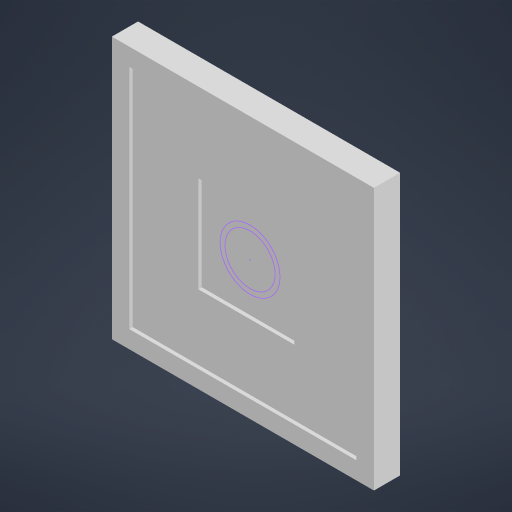
# Autodesk Inventor part: Elbow_Both_Marker_TestFit_V2
Saved by Autodesk Inventor 2024 (Build 280153000, 153)
## iProperties
Created: 2023-06-29
Part Number: Elbow_Both_Marker_TestFit_V2
Material: Generic
Document SubType Name: Modeling
Designer: User
Density: 1 g/cm^3
Appearance: Default
Author: User
Autodesk Inventor part; units mm, degrees
ref_plane "YZ Plane" through (0, 0, 0) normal (1, 0, 0) x (0, 1, 0)
ref_plane "XZ Plane" through (0, 0, 0) normal (0, 1, 0) x (-1, 0, 0)
ref_plane "XY Plane" through (0, 0, 0) normal (0, 0, 1) x (1, 0, 0)
sketch "Sketch4" plane through (0, 0, 0) normal (0, 0, 1) x (1, 0, 0)
  line L0 (0, 0) -> (150, 0)
  line L1 (150, 0) -> (150, 150)
  line L2 (150, 150) -> (0, 150)
  line L3 (0, 150) -> (0, 0)
  dimension "d34" = 150
  dimension "d35" = 150
  constraints: 8 end point, 2 parallel, 1 horizontal, 1 perpendicular
  measures "d34" distance of L2.end L1.end
  measures "d35" distance of L1.end L0.end
extrude "Extrusion4" add sketch "Sketch4" along normal blind 10
sketch "Sketch5" plane through (0, 0, 10) normal (0, 0, 1) x (1, 0, 0)
  line L0 (10, 10) -> (140, 10)
  line L1 (140, 10) -> (140, 140)
  line L2 (140, 140) -> (10, 140)
  line L3 (10, 140) -> (10, 10)
  point P0 (0, 0)
  dimension "d38" = 130
  dimension "d39" = 130
  constraints: 8 end point, 2 parallel, 1 horizontal, 1 perpendicular
  measures "d38" distance of L2.end L1.end
  measures "d39" distance of L1.end L0.end
extrude "Extrusion5" cut sketch "Sketch5" against normal blind 2
sketch "Sketch6" plane through (0, 0, 0) normal (0, 0, -1) x (-1, 0, 0)
  circle A0 centre (-75, 75) radius 14.35
  circle A1 centre (-75, 75) radius 17.15
  line L0 (-147.5, 2.5) -> (-142.5, 2.5)
  line L1 (-142.5, 2.5) -> (-142.5, 7.5)
  line L2 (-142.5, 7.5) -> (-147.5, 7.5)
  line L3 (-147.5, 7.5) -> (-147.5, 2.5)
  line L4 (-2.5, 2.5) -> (-7.5, 2.5)
  line L5 (-7.5, 2.5) -> (-7.5, 7.5)
  line L6 (-7.5, 7.5) -> (-2.5, 7.5)
  line L7 (-2.5, 7.5) -> (-2.5, 2.5)
  line L8 (-147.5, 147.5) -> (-142.5, 147.5)
  line L9 (-142.5, 147.5) -> (-142.5, 142.5)
  line L10 (-142.5, 142.5) -> (-147.5, 142.5)
  line L11 (-147.5, 142.5) -> (-147.5, 147.5)
  line L12 (-2.5, 147.5) -> (-7.5, 147.5)
  line L13 (-7.5, 147.5) -> (-7.5, 142.5)
  line L14 (-7.5, 142.5) -> (-2.5, 142.5)
  line L15 (-2.5, 142.5) -> (-2.5, 147.5)
  point P0 (0, 0)
  dimension "d42" = 28.7
  dimension "d43" = 34.3
  dimension "d46" = 5
  dimension "d47" = 5
  dimension "d48" = 5
  dimension "d49" = 5
  dimension "d50" = 5
  dimension "d51" = 5
  dimension "d52" = 5
  dimension "d53" = 5
  constraints: 32 end point, 8 parallel, 4 horizontal, 4 perpendicular, 2 centre point, 1 coincident
  measures "d42" diameter of A0
  measures "d43" diameter of A1
  measures "d46" distance of L2.end L1.end
  measures "d47" distance of L1.end L0.end
  measures "d48" distance of L5.end L6.end
  measures "d49" distance of L4.end L5.end
  measures "d50" distance of L9.end L10.end
  measures "d51" distance of L8.end L9.end
  measures "d52" distance of L14.end L13.end
  measures "d53" distance of L13.end L12.end
extrude "Extrusion7" cut sketch "Sketch6" against normal blind 5
sketch "Sketch7" plane through (0, 0, 8) normal (0, 0, 1) x (1, 0, 0)
  line L0 (47.5, 102.5) -> (102.5, 102.5)
  line L1 (102.5, 102.5) -> (102.5, 47.5)
  line L2 (102.5, 47.5) -> (47.5, 47.5)
  line L3 (47.5, 47.5) -> (47.5, 102.5)
  point P0 (0, 0)
  dimension "d58" = 55
  dimension "d59" = 55
  constraints: 8 end point, 2 parallel, 1 horizontal, 1 perpendicular
  measures "d58" distance of L1.end L2.end
  measures "d59" distance of L0.end L1.end
extrude "Extrusion8" cut sketch "Sketch7" against normal blind 2
sketch "Sketch9" plane through (0, 0, 6) normal (0, 0, 1) x (1, 0, 0)
  line L0 (47.5, 47.5) -> (47.5, 102.5) projected
  line L1 (47.5, 47.5) -> (102.5, 47.5)
  line L2 (102.5, 47.5) -> (102.5, 102.5)
  line L3 (102.5, 102.5) -> (47.5, 102.5)
  line L4 (47.5, 102.5) -> (47.5, 47.5)
  point P0 (0, 0)
  dimension "d68" = 55
  dimension "d69" = 55
  constraints: 8 end point, 2 parallel, 1 horizontal, 1 perpendicular
  measures "d68" distance of L3.end L2.end
  measures "d69" distance of L2.end L1.end
extrude "Extrusion10" add sketch "Sketch9" along normal blind 2
sketch "Sketch10" plane through (0, 0, 8) normal (0, 0, 1) x (1, 0, 0)
  line L0 (37.5, 37.5) -> (112.5, 37.5) projected
  line L1 (112.5, 37.5) -> (112.5, 112.5) projected
  line L2 (37.5, 37.5) -> (112.5, 37.5)
  line L3 (112.5, 37.5) -> (112.5, 112.5)
  line L4 (112.5, 112.5) -> (37.5, 112.5)
  line L5 (37.5, 112.5) -> (37.5, 37.5)
  point P0 (0, 0)
  dimension "d72" = 75
  dimension "d73" = 75
  constraints: 8 end point, 2 parallel, 1 horizontal, 1 perpendicular
  measures "d72" distance of L4.end L1.end
  measures "d73" distance of L1.end L2.end
extrude "Extrusion11" add sketch "Sketch10" along normal blind 5
sketch "Sketch11" plane through (0, 0, 13) normal (0, 0, 1) x (1, 0, 0)
  line L0 (47.5, 47.5) -> (102.5, 47.5)
  line L1 (102.5, 47.5) -> (102.5, 102.5)
  line L2 (102.5, 102.5) -> (47.5, 102.5)
  line L3 (47.5, 102.5) -> (47.5, 47.5)
  point P0 (0, 0)
  dimension "d76" = 55
  dimension "d77" = 55
  constraints: 8 end point, 2 parallel, 1 horizontal, 1 perpendicular
  measures "d76" distance of L2.end L1.end
  measures "d77" distance of L1.end L0.end
extrude "Extrusion12" cut sketch "Sketch11" against normal blind 2
sketch "Sketch12" plane through (0, 0, 11) normal (0, 0, 1) x (1, 0, 0)
  circle A0 centre (75, 75) radius 14.35
  circle A1 centre (75, 75) radius 17.15
  point P0 (0, 0)
  constraints: 2 centre point, 1 coincident
sketch "Sketch13" plane through (0, 0, 8) normal (0, 0, 1) x (1, 0, 0)
  line L0 (140, 140) -> (140, 10) projected
  line L1 (10, 140) -> (140, 140)
  line L2 (140, 140) -> (140, 10)
  line L3 (140, 10) -> (10, 10)
  line L4 (10, 10) -> (10, 140)
  line L5 (37.5, 37.5) -> (37.5, 112.5) projected
  line L6 (112.5, 112.5) -> (112.5, 37.5) projected
  line L7 (37.5, 112.5) -> (112.5, 112.5)
  line L8 (112.5, 112.5) -> (112.5, 37.5)
  line L9 (112.5, 37.5) -> (37.5, 37.5)
  line L10 (37.5, 37.5) -> (37.5, 112.5)
  point P0 (0, 0)
  constraints: 16 end point, 4 parallel, 2 horizontal, 2 perpendicular
extrude "Extrusion13" add sketch "Sketch13" along normal blind 5
sketch "Sketch15" plane through (0, 0, 10) normal (0, 0, 1) x (1, 0, 0)
  line L0 (0, 0) -> (150, 0)
  line L1 (150, 0) -> (150, 150)
  line L2 (150, 150) -> (0, 150)
  line L3 (0, 150) -> (0, 0)
  line L4 (10, 140) -> (10, 10) projected
  line L5 (10, 140) -> (140, 140)
  line L6 (140, 140) -> (140, 10)
  line L7 (140, 10) -> (10, 10)
  line L8 (10, 10) -> (10, 140)
  dimension "d86" = 150
  dimension "d87" = 150
  dimension "d88" = 130
  dimension "d89" = 130
  constraints: 16 end point, 4 parallel, 2 horizontal, 2 perpendicular
  measures "d86" distance of L2.end L1.end
  measures "d87" distance of L1.end L0.end
  measures "d88" distance of L6.end L7.end
  measures "d89" distance of L5.end L6.end
extrude "Extrusion14" add sketch "Sketch15" along normal blind 5
body "Solid2"
